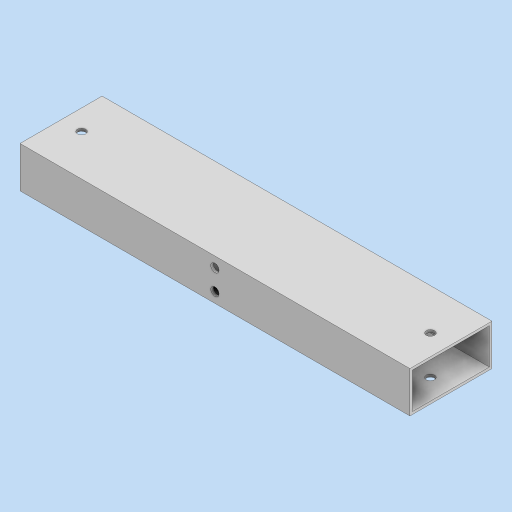
# Autodesk Inventor part: 2inTubeBase
Saved by Autodesk Inventor 2024 (Build 280153000, 153)
## iProperties
Created: 2024-01-10
Part Number: 2inTubeBase
Material: Generic
Document SubType Name: Modeling
Designer: megan
Density: 1 g/cm^3
Appearance: Default
Author: megan
Autodesk Inventor part; units mm, degrees
ref_plane "YZ Plane" through (0, 0, 0) normal (1, 0, 0) x (0, 1, 0)
ref_plane "XZ Plane" through (0, 0, 0) normal (0, 1, 0) x (-1, 0, 0)
ref_plane "XY Plane" through (0, 0, 0) normal (0, 0, 1) x (1, 0, 0)
sketch "Sketch1" plane through (0, 0, 0) normal (1, 0, 0) x (0, 1, 0)
  line L0 (0, 0) -> (25.4, 0)
  line L1 (25.4, 0) -> (25.4, -50.8)
  line L2 (25.4, -50.8) -> (0, -50.8)
  line L3 (0, -50.8) -> (0, 0)
  line L4 (23.8125, -1.5875) -> (1.5875, -1.5875)
  line L5 (1.5875, -1.5875) -> (1.5875, -49.2125)
  line L6 (1.5875, -49.2125) -> (23.8125, -49.2125)
  line L7 (23.8125, -49.2125) -> (23.8125, -1.5875)
  dimension "d0" = 25.4
  dimension "d1" = 50.8
  dimension "d2" = 1.5875
  constraints: 16 end point, 4 parallel, 2 perpendicular, 1 horizontal, 3 other
  measures "d0" distance of L1.end L2.end
  measures "d1" distance of L0.end L1.end
  measures "d2" distance between parallel lines of L0 L4
extrude "Extrusion1" add sketch "Sketch1" along normal blind 241.3
sketch "Sketch2" plane through (0, 25.4, 0) normal (0, 1, 0) x (1, 0, 0)
  line L0 (0, 50.8) -> (0, 0) projected
  line L1 (0, 0) -> (241.3, 0) projected
  line L2 (241.3, 50.8) -> (241.3, 0) projected
  line L3 (0, 50.8) -> (241.3, 50.8) projected
  circle A0 centre (12.7, 25.4) radius 2.5781
  circle A1 centre (228.6, 25.4) radius 2.5781
  point P0 (0, 0)
  dimension "d5" = 5.1562
  dimension "d6" = 12.7
  dimension "d7" = 5.1562
  dimension "d8" = 12.7
  dimension "d9" = 25.4
  dimension "d10" = 25.4
  constraints: 2 centre point
  measures "d5" diameter of A0
  measures "d6" distance from line of L0 A0.centre
  measures "d7" diameter of A1
  measures "d8" distance from line of L2 A1.centre
  measures "d9" distance from line of A0.centre L3
  measures "d10" distance from line of L1 A1.centre
extrude "Extrusion2" cut sketch "Sketch2" against normal blind 25.4 contours A0 | A1
sketch "Sketch3" plane through (0, 0, 0) normal (0, 0, 1) x (1, 0, 0)
  line L0 (0, 25.4) -> (0, 0) projected
  line L1 (0, 0) -> (241.3, 0) projected
  line L2 (241.3, 25.4) -> (241.3, 0) projected
  line L3 (0, 25.4) -> (241.3, 25.4) projected
  circle A0 centre (120.65, 19.05) radius 2.5781
  circle A1 centre (120.65, 6.35) radius 2.5781
  dimension "d13" = 5.1562
  dimension "d14" = 5.1562
  dimension "d15" = 120.65
  dimension "d16" = 120.65
  dimension "d17" = 6.35
  dimension "d18" = 6.35
  constraints: 2 centre point
  measures "d13" diameter of A0
  measures "d14" diameter of A1
  measures "d15" distance from line of L2 A0.centre
  measures "d16" distance from line of L2 A1.centre
  measures "d17" distance from line of L1 A1.centre
  measures "d18" distance from line of L3 A0.centre
extrude "Extrusion3" cut sketch "Sketch3" against normal blind 241.3 contours A0 | A1
body "Solid1"
